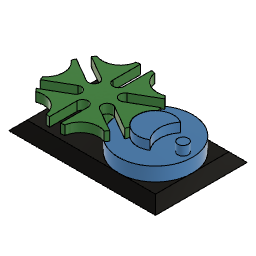
Geneva drive (Autodesk Fusion 360 design; units mm, degrees)
Autodesk Fusion 360 part; units mm, degrees
note: some values were not read from the file. Set by a fixed rule: which sketch regions a step uses.
sketch "down" plane through (0, 0, 0) normal (0, 0, 1) x (1, 0, 0) in component "Base"
  line L0 (0, 50) -> (-80, 50)
  line L1 (-80, 50) -> (-80, -50)
  line L2 (-80, -50) -> (0, -50)
  line L3 (0, 50) -> (80, 50)
  line L4 (80, 50) -> (80, -50)
  line L5 (80, -50) -> (0, -50)
  dimension "d5" = 50
  dimension "d6" = 80
  dimension "d7" = 100
  constraint perpendicular L0 L1
  constraint perpendicular L1 L2
  measures "d5" distance of origin L0.start
  measures "d6" distance of L0.start L0.end
  measures "d7" distance of L0.end L1.end
ref_plane "WorkPlane1" through (0, 0, 10) normal (0, 0, 1) x (1, 0, 0) in component "Base"
sketch "up" plane through (0, 0, 10) normal (0, 0, 1) x (1, 0, 0) in component "Base"
  line L0 (-70, 40) -> (-70, -40)
  line L1 (-70, -40) -> (70, -40)
  line L2 (70, -40) -> (70, 40)
  line L3 (70, 40) -> (-70, 40)
  circle A0 centre (-30, 0) radius 7.5
  circle A1 centre (30, 0) radius 7.5
  dimension "d9" = 15
  dimension "d10" = 15
  constraint vertical L0
  constraint perpendicular L0 L1
  constraint perpendicular L1 L2
  constraint perpendicular L0 L3
  measures "d9" diameter of A0
  measures "d10" diameter of A1
loft "Loft1" add profiles "down", "up" section 1 section 2 makes body 1 in component "Base"
extrude "Extrude1" cut sketch "up" against normal blind 10 contours A0 bodies 1 in component "Base"
extrude "Extrude2" cut sketch "up" against normal blind 10 contours A1 bodies 1 in component "Base"
sketch "holder" plane through (0, 0, 0) normal (0, 0, 1) x (1, 0, 0) in component "Crank"
  circle A0 centre (30, 0) radius 7.5
  dimension "d15" = 15
  measures "d15" diameter of A0
extrude "Extrude1'" add sketch "holder" along normal blind 10 separate body makes body 2 in component "Crank"
move_face "OffsetFaces1" offset -0.3 1 faces at (37.4907, -0.3738, 6.6667) on bodies 2 in component "Crank"
sketch "crank" plane through (0, 0, 10) normal (0, 0, 1) x (1, 0, 0) in component "Crank"
  circle A0 centre (30, 0) radius 40.34
  dimension "d19" = 80.68
  measures "d19" diameter of A0
extrude "Extrude2'" add sketch "crank" along normal blind 15 bodies 2 in component "Crank"
sketch "model" plane through (0, 0, 25) normal (0, 0, 1) x (-1, 0, 0) in component "Crank"
  circle A0 centre (-30, 0) radius 40.34
  arc A1 (-41.1037, -16.6345) -> (-41.1037, 16.6345) centre (-30, 0) ccw
  arc A2 (-41.1037, -16.6345) -> (-41.1037, 16.6345) centre (-60.06, 0) ccw
  circle A3 centre (-60.06, 0) radius 6
  dimension "d22" = 40
  dimension "d23" = 30.06
  dimension "d24" = 50.44
  dimension "d25" = 12
  dimension "d26" = 30.06
  constraint concentric A0 A1
  measures "d22" diameter of A1
  measures "d23" distance of A0.centre A2.centre
  measures "d24" diameter of A2
  measures "d25" diameter of A3
  measures "d26" distance of A0.centre A2.centre
extrude "Extrude3" add sketch "model" along normal blind 10 contours A1 A2 | A3 bodies 2 in component "Crank"
sketch "holder (2)" plane through (0, 0, 0) normal (0, 0, 1) x (1, 0, 0) in component "Wheel"
  circle A0 centre (-30, 0) radius 7.5
  dimension "d29" = 15
  measures "d29" diameter of A0
extrude "Extrude1''" add sketch "holder (2)" along normal blind 10 separate body makes body 3 in component "Wheel"
move_face "OffsetFaces1'" offset -0.3 1 faces at (-22.5093, -0.3738, 6.6667) on bodies 3 in component "Wheel"
sketch "wheel" plane through (0, 0, 10) normal (0, 0, 1) x (1, 0, 0) in component "Wheel"
  line L0 (-36, 19.6387) -> (-36, 49.6387)
  line L1 (-24, 19.6387) -> (-24, 49.6387)
  arc A0 (-36, 19.6387) -> (-24, 19.6387) centre (-30, 19.6387) ccw
  line L2 (-50.0076, 4.6232) -> (-75.9884, 19.6232)
  arc A1 (-50.0076, 4.6232) -> (-44.0076, 15.0155) centre (-47.0076, 9.8193) ccw
  line L3 (-44.0076, 15.0155) -> (-69.9884, 30.0155)
  line L4 (-44.0076, -15.0155) -> (-69.9884, -30.0155)
  arc A2 (-44.0076, -15.0155) -> (-50.0076, -4.6232) centre (-47.0076, -9.8193) ccw
  line L5 (-50.0076, -4.6232) -> (-75.9884, -19.6232)
  line L6 (-24, -19.6387) -> (-24, -49.6387)
  arc A3 (-24, -19.6387) -> (-36, -19.6387) centre (-30, -19.6387) ccw
  line L7 (-36, -19.6387) -> (-36, -49.6387)
  line L8 (-9.9924, -4.6232) -> (15.9884, -19.6232)
  arc A4 (-9.9924, -4.6232) -> (-15.9924, -15.0155) centre (-12.9924, -9.8193) ccw
  line L9 (-15.9924, -15.0155) -> (9.9884, -30.0155)
  line L10 (-15.9924, 15.0155) -> (9.9884, 30.0155)
  arc A5 (-15.9924, 15.0155) -> (-9.9924, 4.6232) centre (-12.9924, 9.8193) ccw
  line L11 (-9.9924, 4.6232) -> (15.9884, 19.6232)
  arc A6 (17.5, 15.6125) -> (17.5, -15.6125) centre (30, 0) ccw
  arc A7 (-19.7708, 48.9425) -> (7.2708, 33.33) centre (0, 51.9615) ccw
  arc A8 (-67.2708, 33.33) -> (-40.2292, 48.9425) centre (-60, 51.9615) ccw
  arc A9 (-77.5, -15.6125) -> (-77.5, 15.6125) centre (-90, 0) ccw
  arc A10 (-40.2292, -48.9425) -> (-67.2708, -33.33) centre (-60, -51.9615) ccw
  arc A11 (7.2708, -33.33) -> (-19.7708, -48.9425) centre (0, -51.9615) ccw
  arc A12 (9.9884, 30.0155) -> (7.2708, 33.33) centre (-30, 0) ccw
  arc A13 (-19.7708, 48.9425) -> (-24, 49.6387) centre (-30, 0) ccw
  arc A14 (-36, 49.6387) -> (-40.2292, 48.9425) centre (-30, 0) ccw
  arc A15 (-67.2708, 33.33) -> (-69.9884, 30.0155) centre (-30, 0) ccw
  arc A16 (-75.9884, 19.6232) -> (-77.5, 15.6125) centre (-30, 0) ccw
  arc A17 (-77.5, -15.6125) -> (-75.9884, -19.6232) centre (-30, 0) ccw
  arc A18 (-69.9884, -30.0155) -> (-67.2708, -33.33) centre (-30, 0) ccw
  arc A19 (-40.2292, -48.9425) -> (-36, -49.6387) centre (-30, 0) ccw
  arc A20 (-24, -49.6387) -> (-19.7708, -48.9425) centre (-30, 0) ccw
  arc A21 (7.2708, -33.33) -> (9.9884, -30.0155) centre (-30, 0) ccw
  arc A22 (15.9884, -19.6232) -> (17.5, -15.6125) centre (-30, 0) ccw
  arc A23 (17.5, 15.6125) -> (15.9884, 19.6232) centre (-30, 0) ccw
  dimension "d33" = 100
  dimension "d34" = 12
  dimension "d35" = 30
  dimension "d36" = 30
  dimension "d38" = 360
  dimension "d39" = 40
  dimension "d40" = 60
  dimension "d42" = 360
  constraint vertical L0
  constraint vertical L1
  constraint concentric A14 A16
  constraint concentric A16 A18
  constraint concentric A18 A20
  constraint concentric A20 A22
  constraint concentric A12 A22
  constraint coincident A6.start A22
  constraint concentric A12 A13
  constraint concentric A14 A15
  constraint concentric A16 A17
  constraint concentric A18 A19
  constraint concentric A20 A21
  constraint concentric A22 A23
  measures "d33" diameter of A14
  measures "d34" diameter of A0
  measures "d35" distance of L0.end L0.start
  measures "d36" distance of L1.end L1.start
  measures "d39" diameter of A6
  measures "d40" distance of A12.centre A6.centre
sketch "top holder" plane through (0, 0, 10) normal (0, 0, 1) x (-1, 0, 0) in component "Wheel"
  circle A0 centre (30, 0) radius 7.2
  circle A1 centre (30, 0) radius 10
extrude "Extrude2''" add sketch "top holder" along normal blind 15 contours A0 | A1 bodies 3 in component "Wheel"
extrude "Extrude3'" add sketch "wheel" along normal blind 10 from surface at 15 bodies 3 in component "Wheel"
move_face "OffsetFaces2" offset -0.3 1 faces at (40.2646, -17.165, 31.6667) on bodies 2 in component "Crank"
move_face "OffsetFaces3" offset -0.3 1 faces at (35.2885, 4.735, 31.6667) on bodies 2 in component "Crank"
move_face "OffsetFaces4" offset -0.3 1 faces at (54.0675, 0.2991, 31.6667) on bodies 2 in component "Crank"
component "Base" placed x (1, 0, 0) y (0, 1, 0) z (0, 0, 1) at (0, 0, 0)
component "Crank" placed x (1, 0, 0) y (0, 1, 0) z (0, 0, 1) at (0, 0, 0)
component "Wheel" placed x (1, 0, 0) y (0, 1, 0) z (0, 0, 1) at (0, 0, 0)
named bodies: "Base", "Crank", "Wheel"
